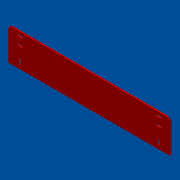
# Autodesk Inventor part: SM-S02
Saved by Autodesk Inventor 2012 SP1 (Build 160190100, 190)
## iProperties
Created: 2011-10-21
Part Number: SM-S02
Material: Steel, Mild
Document SubType Name: Modeling
Designer: ERF
Mass: 859.268 g
Surface Area: 672.796 cm^2
Volume: 109.322 cm^3
Density: 7.86 g/cm^3
Stock Number: SM-S02
Description: 400mm x 80mm 10ga laser cut plate
Vendor: Shapeoko
Project: Shapeoko
Title: Front/Back Plate
Author: ERF
Autodesk Inventor part; units mm, degrees
ref_plane "YZ Plane" through (0, 0, 0) normal (1, 0, 0) x (0, 1, 0)
ref_plane "XZ Plane" through (0, 0, 0) normal (0, 1, 0) x (-1, 0, 0)
ref_plane "XY Plane" through (0, 0, 0) normal (0, 0, 1) x (1, 0, 0)
sketch "Sketch1" plane through (0, 0, 0) normal (0, 0, 1) x (1, 0, 0)
  line L0 (0, 80) -> (400, 80)
  line L1 (400, 80) -> (400, 0)
  line L2 (400, 0) -> (0, 0)
  line L3 (0, 0) -> (0, 80)
  dimension "d0" = 80
  dimension "d1" = 400
  constraints: 8 end point, 2 parallel, 1 horizontal, 1 perpendicular
  measures "d0" distance of L0.end L1.end
  measures "d1" distance of L0.start L0.end
extrude "Extrusion1" add sketch "Sketch1" along normal blind 3.4163
sketch "Sketch2" plane through (0, 0, 3.4163) normal (0, 0, 1) x (1, 0, 0)
  line L0 (0, 80) -> (400, 80) projected
  arc A0 (23.9, 72.5) -> (23.9, 67.5) centre (23.9, 70) ccw
  arc A1 (33.9, 67.5) -> (33.9, 72.5) centre (33.9, 70) ccw
  line L1 (23.9, 72.5) -> (33.9, 72.5)
  line L2 (23.9, 67.5) -> (33.9, 67.5)
  dimension "d7" = 5
  dimension "d8" = 10
  dimension "d9" = 5
  dimension "d10" = 10
  constraints: 4 end point, 4 point on circle, 3 tangent, 2 centre point, 1 parallel
  measures "d7" diameter of A0
  measures "d8" distance from line of L0 A0.centre
  measures "d9" diameter of A1
  measures "d10" distance from line of L0 A1.centre
extrude "Extrusion2" cut sketch "Sketch2" against normal through all
pattern_linear "Rectangular Pattern1" count 2 spacing 342.2 along (1, 0, 0) count 2 spacing 20 along (0, -1, 0) of "Extrusion2"
fillet "Fillet1" radius 10 2 edges at (400, 80, 1.7082) (0, 80, 1.7082)
sketch "Sketch3" plane through (0, 0, 3.4163) normal (0, 0, 1) x (1, 0, 0)
  line L0 (0, 0) -> (0, 70) projected
  line L1 (400, 0) -> (0, 0) projected
  arc A0 (31.4, 20) -> (26.4, 20) centre (28.9, 20) ccw
  arc A1 (26.4, 10) -> (31.4, 10) centre (28.9, 10) ccw
  line L2 (26.4, 20) -> (26.4, 10)
  line L3 (31.4, 20) -> (31.4, 10)
  dimension "d22" = 5
  dimension "d23" = 5
  dimension "d24" = 10
  dimension "d25" = 10
  dimension "d26" = 28.9
  dimension "d27" = 28.9
  constraints: 4 end point, 4 point on circle, 2 centre point, 2 tangent
  measures "d22" diameter of A0
  measures "d23" diameter of A1
  measures "d24" distance of A0.centre A1.centre
  measures "d25" distance from line of L1 A1.centre
  measures "d26" distance from line of L0 A0.centre
  measures "d27" distance from line of L0 A1.centre
extrude "Extrusion3" cut sketch "Sketch3" against normal through all
pattern_linear "Rectangular Pattern2" count 2 spacing 342.2 along (1, 0, 0) of "Extrusion3"
equation "\"d8\" = d6"
equation "\"d10\" = d6"
equation "\"d23\" = d22"
equation "\"d27\" = d26"
equation "\"d6\" = 10"
body "Solid1"
